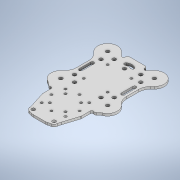
# Autodesk Inventor part: Kauri mid plate V3
Saved by Autodesk Inventor 2020 (Build 240168000, 168)
## iProperties
Created: 2022-08-18
Part Number: Kauri mid plate V3
Material: Generic
Document SubType Name: Modeling
Designer: Steven
Density: 1 g/cm^3
Appearance: Default
Author: Steven
Autodesk Inventor part; units mm, degrees
ref_plane "YZ Plane" through (0, 0, 0) normal (1, 0, 0) x (0, 1, 0)
ref_plane "XZ Plane" through (0, 0, 0) normal (0, 1, 0) x (-1, 0, 0)
ref_plane "XY Plane" through (0, 0, 0) normal (0, 0, 1) x (1, 0, 0)
sketch "Sketch1" plane through (0, 0, 0) normal (0, 1, 0) x (-1, 0, 0)
  arc A0 (24.9, 14.1574) -> (29.1, 14.1574) centre (27, 14.1574) ccw
  line L0 (29.1, 14.1574) -> (29.1, 29.1574)
  arc A1 (29.1, 29.1574) -> (24.9, 29.1574) centre (27, 29.1574) ccw
  line L1 (24.9, 29.1574) -> (24.9, 14.1574)
  arc A2 (4.1506, -4.0991) -> (2.1786, -4.5905) centre (5.0833, -12.0445) ccw
  arc A3 (-2.1786, -4.5905) -> (2.1786, -4.5905) centre (0, 1) ccw
  arc A4 (-2.1786, -4.5905) -> (-4.1506, -4.0991) centre (-5.0833, -12.0445) ccw
  arc A5 (-4.1506, -4.0991) -> (-5.5527, -7.7082) centre (-4.3837, -6.0855) ccw
  arc A6 (-5.5527, -7.7082) -> (5.5527, -7.7082) centre (0, 0) ccw
  arc A7 (5.5527, -7.7082) -> (4.1506, -4.0991) centre (4.3837, -6.0855) ccw
  line L2 (-24.9, 29.1574) -> (-24.9, 14.1574)
  arc A8 (-29.1, 14.1574) -> (-24.9, 14.1574) centre (-27, 14.1574) ccw
  line L3 (-29.1, 14.1574) -> (-29.1, 29.1574)
  arc A9 (-24.9, 29.1574) -> (-29.1, 29.1574) centre (-27, 29.1574) ccw
  ellipse E0 centre (7.3196, 102.715) end of major axis (13.9835, 105.6762) minor radius 6.4402 (10.2387, 108.9524) -> (7.9784, 109.3033) ccw
  line L4 (7.9784, 109.3033) -> (-7.9784, 109.3033)
  ellipse E1 centre (-7.3196, 102.715) end of major axis (-0.6557, 99.7539) minor radius 6.4402 (-7.9784, 109.3033) -> (-10.2387, 108.9524) ccw
  arc A10 (-14.0587, 108.0035) -> (-10.2387, 108.9524) centre (-18.8823, 135.5849) ccw
  arc A11 (-14.0587, 108.0035) -> (-17.7444, 104.1628) centre (-13.2835, 103.5708) ccw
  arc A12 (-18.815, 99.3694) -> (-17.7444, 104.1628) centre (-45.5011, 107.8461) ccw
  line L5 (-18.815, 99.3694) -> (-24.7592, 80.6562)
  arc A13 (-24.7592, 80.6562) -> (-24.9, 79.748) centre (-21.9, 79.748) ccw
  line L6 (-24.9, 79.748) -> (-24.9, 68.8185)
  arc A14 (-27.8412, 67.0538) -> (-24.9, 68.8185) centre (-26.9, 68.8185) ccw
  arc A15 (-27.8412, 67.0538) -> (-30.3028, 66.5886) centre (-28.7824, 65.2891) ccw
  arc A16 (-34.9925, 63.1171) -> (-30.3028, 66.5886) centre (-40.1848, 75.0352) ccw
  arc A17 (-34.9925, 63.1171) -> (-38.8388, 42.8186) centre (-30, 51.6574) ccw
  line L7 (-38.8388, 42.8186) -> (-36.3934, 40.3732)
  arc A18 (-32, 29.7666) -> (-36.3934, 40.3732) centre (-47, 29.7666) ccw
  line L8 (-32, 29.7666) -> (-32, 13.5483)
  arc A19 (-36.3934, 2.9417) -> (-32, 13.5483) centre (-47, 13.5483) ccw
  line L9 (-36.3934, 2.9417) -> (-38.8388, 0.4963)
  arc A20 (-38.8388, 0.4963) -> (-21.1612, -17.1814) centre (-30, -8.3426) ccw
  line L10 (-21.1612, -17.1814) -> (-15.9142, -11.9345)
  arc A21 (-12.5, -13.3487) -> (-15.9142, -11.9345) centre (-14.5, -13.3487) ccw
  line L11 (-12.5, -13.3487) -> (-12.5, -13.8925)
  arc A22 (-12.5, -13.8925) -> (-10, -16.3925) centre (-10, -13.8925) ccw
  line L12 (-10, -16.3925) -> (10, -16.3925)
  arc A23 (10, -16.3925) -> (12.5, -13.8925) centre (10, -13.8925) ccw
  line L13 (12.5, -13.8925) -> (12.5, -13.3487)
  arc A24 (15.9142, -11.9345) -> (12.5, -13.3487) centre (14.5, -13.3487) ccw
  line L14 (15.9142, -11.9345) -> (21.1612, -17.1814)
  arc A25 (21.1612, -17.1814) -> (38.8387, 0.4964) centre (30, -8.3426) ccw
  line L15 (38.8387, 0.4964) -> (36.3934, 2.9417)
  arc A26 (32, 13.5483) -> (36.3934, 2.9417) centre (47, 13.5483) ccw
  line L16 (32, 13.5483) -> (32, 29.7666)
  arc A27 (36.3934, 40.3732) -> (32, 29.7666) centre (47, 29.7666) ccw
  line L17 (36.3934, 40.3732) -> (38.8388, 42.8186)
  arc A28 (38.8388, 42.8186) -> (34.9925, 63.1171) centre (30, 51.6574) ccw
  arc A29 (30.1775, 66.7374) -> (34.9925, 63.1171) centre (40.1848, 75.0352) ccw
  arc A30 (30.1775, 66.7374) -> (27.769, 67.2622) centre (28.6379, 65.4608) ccw
  arc A31 (24.9, 69.0635) -> (27.769, 67.2622) centre (26.9, 69.0635) ccw
  line L18 (24.9, 69.0635) -> (24.9, 79.748)
  arc A32 (24.9, 79.748) -> (24.7592, 80.6562) centre (21.9, 79.748) ccw
  line L19 (24.7592, 80.6562) -> (18.815, 99.3694)
  arc A33 (17.7444, 104.1628) -> (18.815, 99.3694) centre (45.5011, 107.8461) ccw
  arc A34 (17.7444, 104.1628) -> (14.0587, 108.0035) centre (13.2835, 103.5708) ccw
  arc A35 (10.2387, 108.9524) -> (14.0587, 108.0035) centre (18.8823, 135.5849) ccw
  circle A36 centre (15.25, 6.4074) radius 1.5
  circle A37 centre (-15.25, 36.9074) radius 1.5
  circle A38 centre (-15.25, 6.4074) radius 1.5
  circle A39 centre (15.25, 36.9074) radius 1.5
  circle A40 centre (0, 93.6886) radius 1.5
  circle A41 centre (0, 57.6262) radius 1.5
  circle A42 centre (18.0312, 75.6574) radius 1.5
  circle A43 centre (-18.0312, 75.6574) radius 1.5
  circle A44 centre (10, 31.6574) radius 1.5
  circle A45 centre (-10, 11.6574) radius 1.5
  circle A46 centre (10, 11.6574) radius 1.5
  circle A47 centre (-10, 31.6574) radius 1.5
  circle A48 centre (-30, 51.6574) radius 2.275
  circle A49 centre (-25.4558, 4.6869) radius 2.275
  circle A50 centre (30, 51.6574) radius 2.275
  circle A51 centre (25.4558, 4.6869) radius 2.275
  circle A52 centre (25.4558, 38.628) radius 2.275
  circle A53 centre (-16.9706, -3.7984) radius 2.275
  circle A54 centre (-16.9706, 47.1133) radius 2.275
  circle A55 centre (-13.2835, 103.5708) radius 2.275
  circle A56 centre (-30, -8.3426) radius 2.275
  circle A57 centre (16.9706, 47.1133) radius 2.275
  circle A58 centre (16.9706, -3.7984) radius 2.275
  circle A59 centre (30, -8.3426) radius 2.275
  circle A60 centre (0, 0) radius 2.275
  circle A61 centre (-25.4558, 38.628) radius 2.275
  circle A62 centre (13.2835, 103.5708) radius 2.275
  circle A63 centre (-15.25, 60.4074) radius 1.55
  circle A64 centre (15.25, 60.4074) radius 1.55
  circle A65 centre (-10, 65.6574) radius 1.55
  circle A66 centre (10, 65.6574) radius 1.55
  circle A67 centre (10, 85.6574) radius 1.55
  circle A68 centre (-10, 85.6574) radius 1.55
  circle A69 centre (-15.25, 90.9074) radius 1.55
  circle A70 centre (15.25, 90.9074) radius 1.55
  point P0 (10.2387, 108.9524)
  point P1 (7.9784, 109.3033)
  point P2 (-7.9784, 109.3033)
  point P3 (-10.2387, 108.9524)
  point P4 (-14.0587, 108.0035)
  point P5 (-17.7444, 104.1628)
  point P6 (-18.815, 99.3694)
  point P7 (-34.9925, 63.1171)
  point P8 (-38.8388, 42.8186)
  point P9 (15.9142, -11.9345)
  point P10 (21.1612, -17.1814)
  point P11 (32, 13.5483)
  point P12 (32, 29.7666)
  point P13 (34.9925, 63.1171)
  point P14 (30.1775, 66.7374)
  point P15 (27.769, 67.2622)
  point P16 (24.7592, 80.6562)
  point P17 (17.7444, 104.1628)
  point P18 (14.0587, 108.0035)
  point P19 (29.1, 29.1574)
  point P20 (29.1, 14.1574)
  point P21 (24.9, 29.1574)
  point P22 (-2.1786, -4.5905)
  point P23 (2.1786, -4.5905)
  point P24 (-5.5527, -7.7082)
  point P25 (-4.1506, -4.0991)
  point P26 (-24.9, 29.1574)
  constraints: 72 point on circle, 71 centre point, 40 end point, 8 other
extrude "Extrusion1" add sketch "Sketch1" along normal blind 3
sketch "Sketch2" plane through (0, 3, 0) normal (0, 1, 0) x (1, 0, 0)
  circle A0 centre (-10, -11.6574) radius 1.5 projected
  circle A1 centre (-10, -31.6574) radius 1.5 projected
  circle A2 centre (10, -11.6574) radius 1.5 projected
  circle A3 centre (10, -31.6574) radius 1.5 projected
  point P0 (0, 0)
extrude "Extrusion2" add sketch "Sketch2" against normal blind 3
body "Solid1"
